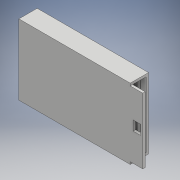
# Autodesk Inventor part: CardBox_4slots
Saved by Autodesk Inventor 2018 (Build 220112000, 112)
## iProperties
Created: 2019-03-10
Part Number: CardBox_4slots
Material: Generic
Document SubType Name: Modeling
Designer: natha
Density: 1 g/cm^3
Appearance: Default
Author: natha
Autodesk Inventor part; units mm, degrees
ref_plane "YZ Plane" through (0, 0, 0) normal (1, 0, 0) x (0, 1, 0)
ref_plane "XZ Plane" through (0, 0, 0) normal (0, 1, 0) x (-1, 0, 0)
ref_plane "XY Plane" through (0, 0, 0) normal (0, 0, 1) x (1, 0, 0)
sketch "Sketch1" plane through (0, 0, 0) normal (0, 0, 1) x (1, 0, 0)
  line L0 (-51.9238, 7.67) -> (40.5487, 7.67)
  line L1 (50.9762, -5.53) -> (50.9762, -7.53)
  line L2 (50.9762, -7.53) -> (-51.9238, -7.53)
  line L3 (-51.9238, -7.53) -> (-51.9238, 7.67)
  line L4 (-51.9238, 7.67) -> (50.9762, -7.53) construction
  line L5 (50.8142, 7.3691) -> (-51.9238, -7.53) construction
  line L6 (40.55, -5.53) -> (50.9762, -5.53)
  line L7 (40.5487, 5.67) -> (-49.9238, 5.67)
  line L8 (-49.9238, 5.67) -> (-49.9238, 3.42)
  line L9 (-49.9238, 3.42) -> (38.3707, 3.42)
  line L10 (40.5487, 7.67) -> (40.5487, 5.8804)
  line L11 (40.55, -5.53) -> (-49.9238, -5.53)
  line L12 (-49.9238, -5.53) -> (-49.9238, -3.28)
  line L13 (-49.9238, -3.28) -> (38.3707, -3.28)
  line L14 (40.5487, 5.8804) -> (40.5487, 5.67)
  line L15 (38.3707, 2.82) -> (-49.9238, 2.82)
  line L16 (-49.9238, 2.82) -> (-49.9238, 0.57)
  line L17 (-49.9238, 0.57) -> (38.3707, 0.57)
  line L18 (38.3707, 3.42) -> (38.3707, 2.82)
  line L19 (38.3707, -0.03) -> (-49.9238, -0.03)
  line L20 (-49.9238, -0.03) -> (-49.9238, -2.28)
  line L21 (-49.9238, -2.28) -> (38.3707, -2.28)
  line L22 (38.3707, 0.57) -> (38.3707, -0.03)
  line L23 (38.3707, -2.28) -> (38.3707, -3.28)
  point P0 (0, 0)
  dimension "d0" = 102.9
  dimension "d1" = 14.9
  dimension "d3" = 2
  dimension "d4" = 2
  dimension "d5" = 2.25
  dimension "d6" = 2
  dimension "d7" = 2
  dimension "d8" = 2.25
  dimension "d10" = 0.6
  dimension "d11" = 2.25
  dimension "d12" = 2
  dimension "d13" = 0.6
  dimension "d14" = 2.25
  dimension "d15" = 1
  dimension "d16" = 2
  constraints: 48 end point, 15 perpendicular, 4 horizontal, 4 point on line, 3 parallel, 2 vertical
  measures "d0" distance of L1.end L2.end
  measures "d1" distance of L5.start L1.end
  measures "d3" distance between parallel lines of L2 L6
  measures "d4" distance between parallel lines of L7 L0
  measures "d5" distance between parallel lines of L9 L7
  measures "d6" distance between parallel lines of L3 L8
  measures "d7" distance between parallel lines of L3 L12
  measures "d8" distance between parallel lines of L11 L13
  measures "d10" distance between parallel lines of L15 L9
  measures "d11" distance between parallel lines of L17 L15
  measures "d12" distance between parallel lines of L3 L16
  measures "d13" distance between parallel lines of L19 L17
  measures "d14" distance between parallel lines of L21 L19
  measures "d15" distance between parallel lines of L13 L21
  measures "d16" distance between parallel lines of L3 L20
extrude "Extrusion1" add sketch "Sketch1" along normal blind 54.5
sketch "Sketch2" plane through (0, 0, 54.5) normal (0, 0, 1) x (1, 0, 0)
  line L0 (-51.9238, 7.67) -> (40.5487, 7.67) projected
  line L1 (50.9762, -7.53) -> (-51.9238, -7.53) projected
  line L2 (40.5487, 7.67) -> (-51.9238, 7.67)
  line L3 (-51.9238, 7.67) -> (-51.9238, -7.53)
  line L4 (-51.9238, -7.53) -> (40.5487, -7.53)
  line L5 (40.5487, -7.53) -> (40.5487, 7.67)
  point P0 (0, 0)
  constraints: 8 end point, 2 parallel, 1 horizontal, 1 perpendicular
extrude "Extrusion2" add sketch "Sketch2" along normal blind 2
sketch "Sketch3" plane through (0, 0, 0) normal (0, 0, -1) x (-1, 0, 0)
  line L0 (-40.5487, 7.67) -> (-40.5487, 5.67) projected
  line L1 (51.9238, -7.53) -> (51.9238, 7.67) projected
  line L2 (-40.5487, 7.67) -> (51.9238, 7.67)
  line L3 (51.9238, 7.67) -> (51.9238, -7.53)
  line L4 (51.9238, -7.53) -> (-40.5487, -7.53)
  line L5 (-40.5487, -7.53) -> (-40.5487, 7.67)
  point P0 (0, 0)
  constraints: 8 end point, 2 parallel, 1 horizontal, 1 perpendicular
extrude "Extrusion3" add sketch "Sketch3" along normal blind 2
sketch "Sketch4" plane through (40.5487, -7.53, 0) normal (0, -1, 0) x (1, 0, 0)
  line L0 (8.4275, 31.25) -> (2.4275, 31.25)
  line L1 (2.4275, 31.25) -> (2.4275, 23.25)
  line L2 (2.4275, 23.25) -> (8.4275, 23.25)
  line L3 (8.4275, 23.25) -> (8.4275, 31.25)
  line L4 (10.4275, 0) -> (10.4275, 54.5) projected
  line L5 (10.4275, 0) -> (0, 0) projected
  point P0 (-40.5487, 0)
  dimension "d23" = 2
  dimension "d24" = 8
  dimension "d25" = 6
  dimension "d26" = 23.25
  constraints: 8 end point, 2 parallel, 1 horizontal, 1 perpendicular
  measures "d23" distance between parallel lines of L4 L3
  measures "d24" distance between parallel lines of L2 L0
  measures "d25" distance between parallel lines of L3 L1
  measures "d26" distance between parallel lines of L5 L2
extrude "Extrusion4" cut sketch "Sketch4" against normal blind 2
body "Solid1"
